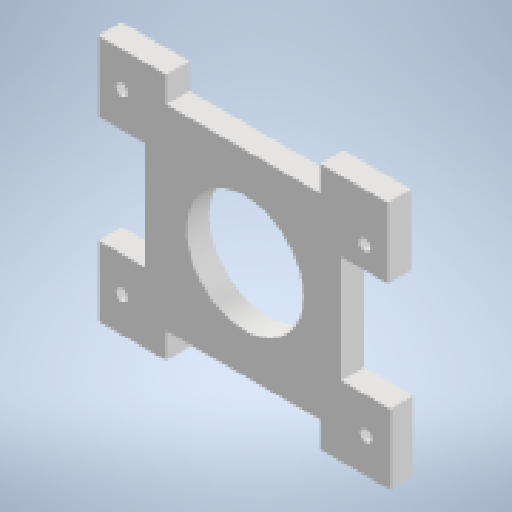
# Autodesk Inventor part: Drzalo_motorja
Saved by Autodesk Inventor 2023 (Build 270158000, 158)
## iProperties
Created: 2022-09-16
Part Number: Drzalo_motorja
Material: Generic
Document SubType Name: Modeling
Designer: simon
Density: 1 g/cm^3
Appearance: Default
Author: simon
Autodesk Inventor part; units mm, degrees
ref_plane "YZ Plane" through (0, 0, 0) normal (1, 0, 0) x (0, 1, 0)
ref_plane "XZ Plane" through (0, 0, 0) normal (0, 1, 0) x (-1, 0, 0)
ref_plane "XY Plane" through (0, 0, 0) normal (0, 0, 1) x (1, 0, 0)
sketch "Sketch2" plane through (0, 0, 0) normal (0, 0, 1) x (1, 0, 0)
  circle A0 centre (4.5, -2.75) radius 1.25 projected
  line L0 (9.5, 7.5) -> (-5, 7.5) projected
  line L1 (-5, 7.5) -> (-5, 2) projected
  line L2 (-5, 2) -> (-0.5, 2) projected
  line L3 (-0.5, 2) -> (-0.5, -7.5) projected
  line L4 (-0.5, -7.5) -> (7.5, -7.5) projected
  line L5 (9.5, -5.5) -> (9.5, 7.5) projected
  circle A1 centre (4.75, -38) radius 1.25 projected
  line L6 (-5, -45.5) -> (8, -45.5) projected
  line L7 (10, -43.5) -> (10, -32.5) projected
  line L8 (8, -30.5) -> (-0.5, -30.5) projected
  line L9 (-0.5, -30.5) -> (-0.5, -40) projected
  line L10 (-0.5, -40) -> (-5, -40) projected
  line L11 (-5, -40) -> (-5, -45.5) projected
  circle A2 centre (-47.5, -38) radius 1.25 projected
  line L12 (-38, -40) -> (-42.5, -40) projected
  line L13 (-42.5, -40) -> (-42.5, -30.5) projected
  line L14 (-42.5, -30.5) -> (-50.5, -30.5) projected
  line L15 (-52.5, -32.5) -> (-52.5, -43.5) projected
  line L16 (-50.5, -45.5) -> (-38, -45.5) projected
  line L17 (-38, -45.5) -> (-38, -40) projected
  circle A3 centre (-47.5, 0) radius 1.25 projected
  line L18 (-42.5, -7.5) -> (-42.5, 2) projected
  line L19 (-42.5, 2) -> (-38, 2) projected
  line L20 (-38, 2) -> (-38, 7.5) projected
  line L21 (-38, 7.5) -> (-50.5, 7.5) projected
  line L22 (-52.5, 5.5) -> (-52.5, -5.5) projected
  line L23 (-50.5, -7.5) -> (-42.5, -7.5) projected
  circle A4 centre (-21.1548, -18.9993) radius 2.5 projected
  circle A5 centre (-21.1548, -18.9993) radius 12.5 projected
  line L24 (-0.5, 2) -> (-42.5, 2)
  line L25 (-42.5, 2) -> (-42.5, -40)
  line L26 (-42.5, -40) -> (-0.5, -40)
  line L27 (-0.5, -40) -> (-0.5, 2)
  arc A6 (-52.5, -5.5) -> (-50.5, -7.5) centre (-50.5, -5.5) ccw projected
  arc A7 (-50.5, 7.5) -> (-52.5, 5.5) centre (-50.5, 5.5) ccw projected
  arc A8 (8, -45.5) -> (10, -43.5) centre (8, -43.5) ccw projected
  arc A9 (10, -32.5) -> (8, -30.5) centre (8, -32.5) ccw projected
  arc A10 (7.5, -7.5) -> (9.5, -5.5) centre (7.5, -5.5) ccw projected
  arc A11 (-52.5, -43.5) -> (-50.5, -45.5) centre (-50.5, -43.5) ccw projected
  arc A12 (-50.5, -30.5) -> (-52.5, -32.5) centre (-50.5, -32.5) ccw projected
  line L28 (9.5, 2) -> (-52.5, 2)
  line L29 (9.5, 2) -> (-52.5, 2)
  point P0 (0, 0)
  constraints: 12 end point, 3 horizontal, 2 parallel, 2 point on line, 1 perpendicular
extrude "Extrusion1" add sketch "Sketch2" along normal blind 5 contours L5 L28 L2 L1 L0 | L5 A10 L4 L3 L28 | L2 L3 L27 L9 L10 L26 L12 L13 L25 L18 L19 L24 | L19 L28 L22 A7 L21 L20 | L18 L23 A6 L22 L28 | L8 A9 L7 A8 L6 L11 L10 L9 | L13 L12 L17 L16 A11 L15 A12 L14
body "Solid1"
